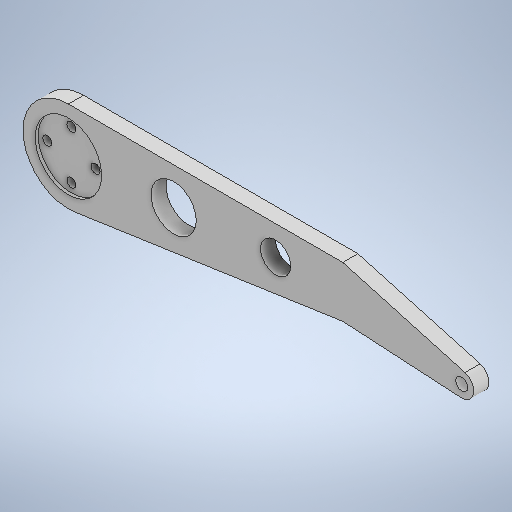
# Autodesk Inventor part: Link1
Saved by Autodesk Inventor 2025 (Build 290162000, 162)
## iProperties
Created: 2026-08-08
Part Number: Link1
Material: Generic
Document SubType Name: Sheet Metal
Designer: MSI
Density: 1 g/cm^3
Sheet Metal Rule: Default_mm
Appearance: Default
Author: MSI
Autodesk Inventor part; units mm, degrees
ref_plane "YZ Plane" through (0, 0, 0) normal (1, 0, 0) x (0, 1, 0)
ref_plane "XZ Plane" through (0, 0, 0) normal (0, 1, 0) x (-1, 0, 0)
ref_plane "XY Plane" through (0, 0, 0) normal (0, 0, 1) x (1, 0, 0)
sketch "Sketch1" plane through (0, 0, 0) normal (0, 0, 1) x (1, 0, 0)
  circle A0 centre (0, 0) radius 11
  arc A1 (0, 15) -> (2.1765, -14.8412) centre (0, 0) ccw
  arc A2 (129.7656, -4.1488) -> (131.0779, 3.6963) centre (129.9999, -0.1557) ccw
  line L0 (131.0779, 3.6963) -> (90.6866, 15)
  line L1 (90.6866, 15) -> (0, 15)
  line L2 (2.1765, -14.8412) -> (90.7092, -1.8575)
  line L3 (90.7092, -1.8575) -> (129.7656, -4.1488)
  circle A3 centre (68.4834, 5.3471) radius 5
  circle A4 centre (34.7617, 2.7142) radius 7.5
  circle A5 centre (129.9999, -0.1557) radius 2
  circle A6 centre (0, 8) radius 1.5
  circle A7 centre (-8, 0) radius 1.5
  circle A8 centre (0, -8) radius 1.5
  circle A9 centre (8, 0) radius 1.5
  dimension "d0" = 22
  dimension "d1" = 30
  dimension "d2" = 8
  dimension "d3" = 130
  dimension "d4" = 15
  dimension "d5" = 10
  dimension "d6" = 4
  dimension "d7" = 3
  dimension "d8" = 8
  dimension "d11" = 360
  constraints: 10 centre point, 8 end point, 4 point on circle, 4 tangent, 3 coincident, 9 other
  measures "d0" diameter of A0
  measures "d1" diameter of A1
  measures "d2" diameter of A2
  measures "d3" distance of A2.centre point (0, 0)
  measures "d4" diameter of A4
  measures "d5" diameter of A3
  measures "d6" diameter of A5
  measures "d7" diameter of A6
  measures "d8" distance of A6.centre point (0, 0)
extrude "Extrusion1" add sketch "Sketch1" along normal blind 5 contours L1 L0 A2 L3 L2 A1
extrude "Extrusion2" add sketch "Sketch1" along normal blind 4 contours A0
equation "\"BendRadius\" = Thickness"
equation "\"BendReliefWidth\" = Thickness"
equation "\"BendReliefDepth\" = 0.5 * Thickness"
equation "\"CornerReliefSize\" = 4 * Thickness"
equation "\"MinimumRemnant\" = 2 * Thickness"
equation "\"TransitionRadius\" = BendRadius"
equation "\"JacobiRadiusSize\" = BendRadius"
equation "\"GapSize\" = Thickness"
equation "\"Thickness\" = 0.5"
body "Solid1"
